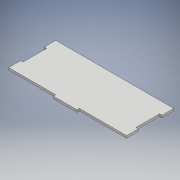
# Autodesk Inventor part: atas
Saved by Autodesk Inventor 2017 (Build 210142000, 142)
## iProperties
Created: 2017-01-17
Part Number: atas
Material: Generic
Document SubType Name: Modeling
Designer: Ghesa Bhakti
Density: 1 g/cm^3
Appearance: Default
Author: Ghesa Bhakti
Autodesk Inventor part; units mm, degrees
ref_plane "YZ Plane" through (0, 0, 0) normal (1, 0, 0) x (0, 1, 0)
ref_plane "XZ Plane" through (0, 0, 0) normal (0, 1, 0) x (-1, 0, 0)
ref_plane "XY Plane" through (0, 0, 0) normal (0, 0, 1) x (1, 0, 0)
sketch "Sketch1" plane through (0, 0, 0) normal (0, 0, 1) x (1, 0, 0)
  line L0 (90, 0) -> (90, -3)
  line L1 (60, -3) -> (60, 0)
  line L2 (0, 60) -> (0, 45)
  line L3 (3, 45) -> (3, 15)
  line L4 (0, 45) -> (3, 45)
  line L5 (3, 15) -> (0, 15)
  line L6 (0, 15) -> (0, 0)
  line L7 (0, 0) -> (60, 0)
  line L8 (90, -3) -> (60, -3)
  line L9 (90, 0) -> (150, 0)
  line L10 (150, 60) -> (0, 60)
  line L11 (150, 15) -> (147, 15)
  line L12 (147, 15) -> (147, 45)
  line L13 (147, 45) -> (150, 45)
  line L14 (150, 0) -> (150, 15)
  line L15 (150, 45) -> (150, 60)
  dimension "d10" = 150
  dimension "d11" = 60
  dimension "d12" = 3
  dimension "d13" = 15
  dimension "d14" = 3
  dimension "d15" = 30
  dimension "d16" = 30
  dimension "d17" = 3
  dimension "d18" = 3
  dimension "d19" = 15
  constraints: 32 end point, 5 horizontal, 3 parallel, 2 perpendicular, 2 vertical
  measures "d10" distance of L7.start L9.end
  measures "d11" distance of L10.end L7.start
  measures "d12" distance of L0.start L8.start
  measures "d13" distance of L10.end L4.start
  measures "d14" distance of L3.end L6.start
  measures "d15" distance of L8.start L8.end
  measures "d16" distance of L12.start L13.start
  measures "d17" distance of L11.start L12.start
  measures "d18" distance of L13.start L15.start
  measures "d19" distance of L9.end L11.start
extrude "Extrusion1" add sketch "Sketch1" along normal blind 3
body "Solid1"
